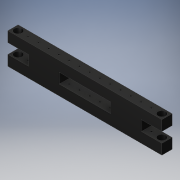
# Autodesk Inventor part: RobotArm Board
Saved by Autodesk Inventor 2018.2 (Build 222227000, 227)
## iProperties
Created: 2018-01-13
Part Number: RobotArm Board
Material: Generic
Document SubType Name: Modeling
Designer: lopez.xavier
Density: 1 g/cm^3
Appearance: Glossy - Black
Author: lopez.xavier
Autodesk Inventor part; units mm, degrees
ref_plane "YZ Plane" through (0, 0, 0) normal (1, 0, 0) x (0, 1, 0)
ref_plane "XZ Plane" through (0, 0, 0) normal (0, 1, 0) x (-1, 0, 0)
ref_plane "XY Plane" through (0, 0, 0) normal (0, 0, 1) x (1, 0, 0)
sketch "Sketch1" plane through (0, 0, 0) normal (0, 0, 1) x (1, 0, 0)
  line L0 (0, 0) -> (381, 0)
  line L1 (381, 0) -> (381, 76.2)
  line L2 (381, 76.2) -> (0, 76.2)
  line L3 (0, 76.2) -> (0, 0)
  dimension "d0" = 381
  dimension "d1" = 76.2
  constraints: 8 end point, 2 parallel, 1 horizontal, 1 perpendicular
  measures "d0" distance of L2.end L1.end
  measures "d1" distance of L0.end L1.end
extrude "Extrusion1" add sketch "Sketch1" along normal blind 25.4
sketch "Sketch7" plane through (0, 0, 25.4) normal (0, 0, 1) x (1, 0, 0)
  line L0 (0, 50.8) -> (50.8, 50.8)
  line L1 (50.8, 50.8) -> (50.8, 25.4)
  line L2 (50.8, 25.4) -> (0, 25.4)
  line L3 (0, 25.4) -> (0, 50.8)
  line L4 (127, 50.8) -> (254, 50.8)
  line L5 (254, 50.8) -> (254, 25.4)
  line L6 (254, 25.4) -> (127, 25.4)
  line L7 (127, 25.4) -> (127, 50.8)
  line L8 (330.2, 50.8) -> (381, 50.8)
  line L9 (381, 50.8) -> (381, 25.4)
  line L10 (381, 25.4) -> (330.2, 25.4)
  line L11 (330.2, 25.4) -> (330.2, 50.8)
  line L12 (381, 76.2) -> (0, 76.2) projected
  line L13 (0, 0) -> (381, 0) projected
  line L14 (0, 76.2) -> (0, 0) projected
  line L15 (381, 0) -> (381, 76.2) projected
  dimension "d34" = 25.4
  dimension "d35" = 25.4
  dimension "d36" = 25.4
  dimension "d37" = 25.4
  dimension "d38" = 0
  dimension "d39" = 0
  dimension "d40" = 76.2
  dimension "d41" = 76.2
  dimension "d42" = 50.8
  dimension "d43" = 50.8
  constraints: 24 end point, 6 parallel, 3 horizontal, 3 perpendicular, 2 point on line
  measures "d34" distance between parallel lines of L12 L0
  measures "d35" distance between parallel lines of L12 L4
  measures "d36" distance between parallel lines of L13 L6
  measures "d37" distance between parallel lines of L13 L10
  measures "d38" distance between parallel lines of L14 L3
  measures "d39" distance between parallel lines of L15 L9
  measures "d40" distance between parallel lines of L11 L5
  measures "d41" distance between parallel lines of L1 L7
  measures "d42" distance of L0.start L0.end
  measures "d43" distance of L8.start L8.end
extrude "Extrusion6" cut sketch "Sketch7" against normal blind 25.4 contours L0 L1 L2 L3 | L9 L10 L11 L8 | L4 L5 L6 L7
sketch "Sketch8" plane through (0, 76.2, 0) normal (0, 1, 0) x (1, 0, 0)
  circle A0 centre (12.7, -12.7) radius 2.3812
  line L0 (381, -25.4) -> (0, -25.4) projected
  circle A1 centre (38.1, -12.7) radius 2.3812
  circle A2 centre (63.5, -12.7) radius 2.3812
  circle A3 centre (88.9, -12.7) radius 2.3812
  circle A4 centre (114.3, -12.7) radius 2.3812
  circle A5 centre (139.7, -12.7) radius 2.3812
  circle A6 centre (165.1, -12.7) radius 2.3812
  circle A7 centre (190.5, -12.7) radius 2.3812
  circle A8 centre (215.9, -12.7) radius 2.3812
  circle A9 centre (241.3, -12.7) radius 2.3812
  circle A10 centre (266.7, -12.7) radius 2.3812
  circle A11 centre (292.1, -12.7) radius 2.3812
  circle A12 centre (317.5, -12.7) radius 2.3812
  line L1 (0, 0) -> (0, -25.4) projected
  circle A13 centre (342.9, -12.7) radius 2.3812
  circle A14 centre (368.3, -12.7) radius 2.3812
  circle A15 centre (368.3, -12.7) radius 9.525
  circle A16 centre (12.7, -12.7) radius 9.525
  dimension "d46" = 4.7625
  dimension "d47" = 12.7
  dimension "d50" = 25.4
  dimension "d55" = 12.7
  dimension "d58" = 19.05
  dimension "d59" = 19.05
  constraints: 17 centre point, 2 coincident, 1 horizontal, 28 other
  measures "d46" diameter of A0
  measures "d47" distance from line of L0 A0.centre
  measures "d50" distance of A0.centre A1.centre
  measures "d55" distance from line of L1 A0.centre
  measures "d58" diameter of A15
  measures "d59" diameter of A16
extrude "Extrusion7" cut sketch "Sketch8" against normal blind 76.2 contours A0 | A1 | A2 | A3 | A4 | A5 | A6 | A7 | A8 | A9 | A10 | A11 | A12 | A13 | A14 | A15 | A16
equation "\"d35\" = d34"
equation "\"d37\" = d36"
body "Solid1"
